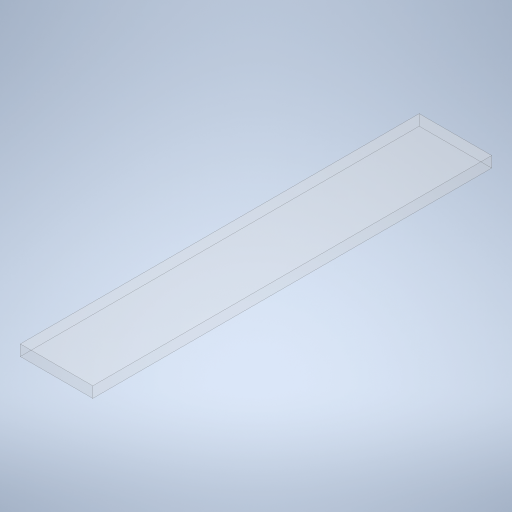
# Autodesk Inventor part: 초음파센서거리측정용아크릴판
Saved by Autodesk Inventor 2024 (Build 280153000, 153)
## iProperties
Created: 2024-04-21
Part Number: 초음파센서거리측정용아크릴판
Material: PMMA 플라스틱
Document SubType Name: Modeling
Designer: kkamin5
Density: 1.188 g/cm^3
Appearance: 폴리카보네이트 - 선명
Mass: 7.8408 g
Surface Area: 51.8 cm^2
Volume: 6.6 cm^3
Author: kkamin5
Autodesk Inventor part; units mm, degrees
ref_plane "YZ Plane" through (0, 0, 0) normal (1, 0, 0) x (0, 1, 0)
ref_plane "XZ Plane" through (0, 0, 0) normal (0, 1, 0) x (-1, 0, 0)
ref_plane "XY Plane" through (0, 0, 0) normal (0, 0, 1) x (1, 0, 0)
sketch "스케치1" plane through (0, 0, 0) normal (0, 1, 0) x (-1, 0, 0)
  line L0 (10, 55) -> (-10, 55)
  line L1 (-10, 55) -> (-10, -55)
  line L2 (-10, -55) -> (10, -55)
  line L3 (10, -55) -> (10, 55)
  point P0 (0, 0)
  dimension "d0" = 20
  dimension "d1" = 110
  dimension "d4" = 55
  dimension "d5" = 10
  constraints: 8 end point, 2 parallel, 1 horizontal, 1 perpendicular
  measures "d0" distance of L1.end L2.end
  measures "d1" distance of L0.end L1.end
  measures "d4" distance from line of point (0, 0) L0
  measures "d5" distance from line of point (0, 0) L3
extrude "돌출1" add sketch "스케치1" along normal blind 3
